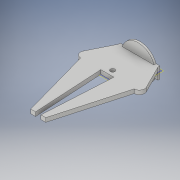
# Autodesk Inventor part: gripper
Saved by Autodesk Inventor 2017 (Build 210142000, 142)
## iProperties
Created: 2017-03-03
Part Number: gripper
Material: Generic
Document SubType Name: Modeling
Designer: Canton
Density: 1 g/cm^3
Appearance: Default
Author: Canton
Autodesk Inventor part; units mm, degrees
ref_plane "YZ Plane" through (0, 0, 0) normal (1, 0, 0) x (0, 1, 0)
ref_plane "XZ Plane" through (0, 0, 0) normal (0, 1, 0) x (-1, 0, 0)
ref_plane "XY Plane" through (0, 0, 0) normal (0, 0, 1) x (1, 0, 0)
sketch "Sketch2" plane through (0, 0, 0) normal (0, 0, 1) x (1, 0, 0)
  line L0 (-24.5, 0) -> (-24.5, 7)
  line L1 (-24.5, 0) -> (-24.5, -7)
  line L2 (-24.5, 7) -> (-19.799, 7)
  line L3 (-24.5, -7) -> (-19.799, -7)
  line L4 (24.5, 7) -> (19.799, 7)
  line L5 (24.5, 0) -> (24.5, 7)
  line L6 (24.5, 0) -> (24.5, -7)
  line L7 (24.5, -7) -> (19.799, -7)
  arc A0 (-19.799, -7) -> (19.799, -7) centre (0, 0) ccw
  arc A1 (19.799, 7) -> (-19.799, 7) centre (0, 0) ccw
  circle A2 centre (0, 0) radius 2.75
  point P0 (0, 0)
  point P1 (0, -4.75)
  point P2 (-27.5, 17.25)
  dimension "d0" = 5.5
  constraints: 16 end point, 4 point on circle, 3 centre point, 2 horizontal, 2 vertical, 1 coincident
  measures "d0" diameter of A2
extrude "Extrusion1" add sketch "Sketch2" along normal blind 2.5
ref_plane "Work Plane1" through (-24.5, -7, 2.5) normal (0, 0, 1) x (1, 0, 0)
sketch "Sketch3" plane through (-24.5, -7, 2.5) normal (0, 0, 1) x (1, 0, 0)
  line L0 (0, 14) -> (49, 14)
  line L1 (49, 14) -> (49, 9)
  line L2 (49, 9) -> (0, 9)
  line L3 (0, 9) -> (0, 14)
  dimension "d3" = 5
  constraints: 8 end point, 2 parallel, 1 horizontal, 1 perpendicular
  measures "d3" distance of L0.end L1.end
extrude "Extrusion2" add sketch "Sketch3" along normal blind 38
ref_plane "Work Plane2" through (-24.5, 2, 40.5) normal (0, -1, 0) x (1, 0, 0)
sketch "Sketch6" plane through (-24.5, 2, 40.5) normal (0, -1, 0) x (1, 0, 0)
  line L0 (0, -40.5) -> (0, -38) projected
  line L1 (-8.6, 0) -> (0, 0)
  line L2 (0, 0) -> (0, -38)
  arc A0 (-8.6, 0) -> (-14.3279, -9.2551) centre (-8.6, -6.4) ccw
  line L3 (0, -38) -> (-14.3279, -9.2551)
  line L4 (49, -40.5) -> (49, 0) projected
  arc A1 (63.3279, -9.2551) -> (57.6, 0) centre (57.6, -6.4) ccw
  line L5 (0, 0) -> (49, 0) projected
  line L6 (49, 0) -> (57.6, 0)
  line L7 (49, -38) -> (63.3279, -9.2551)
  point P0 (24.5, -40.5)
  constraints: 10 end point, 4 point on circle, 3 tangent, 2 centre point, 1 collinear, 1 point on line
extrude "Extrusion5" add sketch "Sketch6" against normal blind 5
sketch "Sketch7" plane through (-24.5, 2, 40.5) normal (0, -1, 0) x (1, 0, 0)
  line L0 (24.5, -6.5) -> (116.5, -6.5) construction
  line L1 (15.25, 85.5) -> (-8.6, 0)
  line L2 (33.75, 85.5) -> (57.6, 0)
  line L3 (15.25, 85.5) -> (21.25, 85.5)
  line L4 (33.75, 85.5) -> (27.75, 85.5)
  line L5 (57.6, 0) -> (32.6, 0)
  line L6 (-8.6, 0) -> (16.4, 0)
  line L7 (21.25, 85.5) -> (16.4, 0)
  line L8 (27.75, 85.5) -> (32.6, 0)
  point P0 (24.5, -40.5)
  constraints: 18 end point, 3 horizontal
sketch "Sketch8" plane through (-24.5, 2, 40.5) normal (0, -1, 0) x (1, 0, 0)
  circle A0 centre (24.5, -6.519) radius 2.75
  point P0 (24.5, -40.5)
  dimension "d35" = 5.5
  constraints: 1 centre point
  measures "d35" diameter of A0
extrude "Extrusion6" add sketch "Sketch7" against normal blind 5
extrude "Extrusion7" cut sketch "Sketch8" against normal blind 5
body "Solid1"
